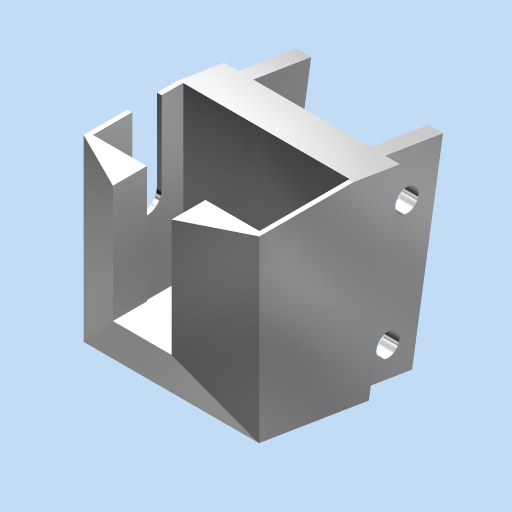
# Autodesk Inventor part: back_mount
Saved by Autodesk Inventor 2024 (Build 280153000, 153)
## iProperties
Created: 2024-02-18
Part Number: back_mount
Material: Aluminum 6061
Document SubType Name: Modeling
Designer: Monesh Ponduri
Density: 2.71 g/cm^3
Appearance: Aluminum - Flat
Author: Monesh Ponduri
## iProperties of the stored document back_mount_3DPrint.ipt
Created: 2024-02-20
Part Number: back_mount_3DPrint
Material: Generic
Document SubType Name: Modeling
Designer: mones
Density: 1 g/cm^3
Appearance: Default
Author: mones
Autodesk Inventor part; units mm, degrees
ref_plane "YZ Plane Vertical Spine" through (0, 0, 0) normal (1, 0, 0) x (0, 1, 0)
ref_plane "XZ Plane Horizontal" through (0, 0, 0) normal (0, 1, 0) x (-1, 0, 0)
ref_plane "XY Plane Vertical Span" through (0, 0, 0) normal (0, 0, 1) x (1, 0, 0)
sketch "Sketch1" plane through (0, 0, 0) normal (1, 0, 0) x (0, 1, 0)
  circle A0 centre (9.6489, 11.4476) radius 2.4892
  line L0 (2.3561, 6.2073) -> (18.2812, 3.5994)
  line L1 (33.7025, 135.9395) -> (135.3025, 135.9395) construction
  line L2 (21.99, 26.2473) -> (-14.84, 26.2473)
  line L3 (4.4085, 18.7403) -> (-20.6576, 22.8451)
  line L4 (-20.6576, 22.8451) -> (-22.71, 10.312)
  line L5 (-22.71, 10.312) -> (2.3561, 6.2073)
  circle A1 centre (-15.4173, 15.5524) radius 2.4892
  line L6 (-14.84, 26.2473) -> (-14.84, 46.5673)
  line L7 (-20.6576, 22.8451) -> (-16.7225, 46.8756)
  line L8 (-16.7225, 46.8756) -> (-14.84, 46.5673)
  line L9 (21.99, 26.2473) -> (18.2812, 3.5994)
  line L10 (20.3336, 16.1325) -> (4.4085, 18.7403)
  dimension "d11" = 12.7
  dimension "d13" = 4.9784
  dimension "d14" = 20.32
  constraints: 22 end point, 3 perpendicular, 2 centre point, 1 horizontal, 1 point on line, 1 vertical
  measures "d11" distance of L3.end L4.end
  measures "d13" diameter of A1
  measures "d14" distance of L2.end L6.end
extrude "Extrusion1" add sketch "Sketch1" along normal blind 3.175
sketch "Sketch2" plane through (0, 0, 0) normal (-1, 0, 0) x (0, 0, 1)
  line L0 (26.2473, 21.99) -> (26.2473, -14.84) projected
  line L1 (3.5994, 18.2812) -> (26.2473, 21.99) projected
  line L2 (26.2473, -14.84) -> (46.5673, -14.84) projected
  line L3 (46.8756, -16.7225) -> (10.312, -22.71) projected
  line L4 (16.1325, 20.3336) -> (22.8451, -20.6576)
  line L5 (16.1325, 20.3336) -> (26.2473, 21.99)
  line L6 (26.2473, 21.5334) -> (26.2473, -14.84)
  line L7 (26.2473, -14.84) -> (46.5673, -14.84)
  line L8 (46.5673, -14.84) -> (46.8756, -16.7225)
  line L9 (46.8756, -16.7225) -> (22.8451, -20.6576)
  constraints: 12 end point, 4 collinear, 3 point on line, 2 perpendicular
extrude "Extrusion2" add sketch "Sketch2" along normal blind 25.4
sketch "Sketch3" plane through (-25.4, 0, 0) normal (-1, 0, 0) x (0, 0, 1)
  line L0 (26.2473, -14.84) -> (26.2473, 21.99) projected
  line L1 (3.5994, 18.2812) -> (16.1325, 20.3336) projected
  line L2 (26.2473, 21.99) -> (16.1325, 20.3336) projected
  line L3 (46.5673, -14.84) -> (26.2473, -14.84) projected
  line L4 (46.8756, -16.7225) -> (46.5673, -14.84) projected
  line L5 (22.8451, -20.6576) -> (46.8756, -16.7225) projected
  line L6 (22.8451, -20.6576) -> (10.312, -22.71) projected
  line L7 (10.312, -22.71) -> (3.5994, 18.2812) projected
  circle A0 centre (15.5524, -15.4173) radius 2.4892 projected
  circle A1 centre (11.4476, 9.6489) radius 2.4892 projected
extrude "Extrusion3" add sketch "Sketch3" along normal blind 3.175
sketch "Sketch4" plane through (-28.575, 0, 0) normal (-1, 0, 0) x (0, 0, 1)
  line L0 (26.2473, 21.99) -> (3.5994, 18.2812) projected
  line L1 (26.2473, -14.84) -> (26.2473, 21.99) projected
  line L2 (46.5673, -14.84) -> (26.2473, -14.84) projected
  line L3 (46.8756, -16.7225) -> (46.5673, -14.84) projected
  line L4 (10.312, -22.71) -> (46.8756, -16.7225) projected
  line L5 (46.8756, -16.7225) -> (46.5673, -14.84) projected
  line L6 (46.5673, -14.84) -> (26.2473, -14.84) projected
  line L7 (26.2473, -14.84) -> (26.2473, 21.99) projected
  line L8 (26.2473, 21.99) -> (3.5994, 18.2812) projected
  line L9 (3.5994, 18.2812) -> (10.312, -22.71) projected
  line L10 (10.312, -22.71) -> (46.8756, -16.7225) projected
  circle A0 centre (11.4476, 9.6489) radius 2.4892 projected
  circle A1 centre (15.5524, -15.4173) radius 2.4892 projected
  line L11 (16.1325, 20.3336) -> (22.8451, -20.6576)
  line L12 (16.1325, 20.3336) -> (26.2473, 21.99)
  line L13 (26.2473, 21.99) -> (26.2473, -14.84)
  line L14 (46.5673, -14.84) -> (26.2473, -14.84)
  line L15 (46.5673, -14.84) -> (46.8756, -16.7225)
  line L16 (46.8756, -16.7225) -> (22.8451, -20.6576)
  constraints: 12 end point, 4 perpendicular, 2 collinear, 1 point on line
extrude "Extrusion4" add sketch "Sketch4" along normal blind 3.175 contours L1 L2 L3 L4 L11 L0
sketch "Sketch5" plane through (3.175, 0, 0) normal (1, 0, 0) x (0, 0, -1)
  line L0 (-22.8451, -20.6576) -> (-16.1325, 20.3336) projected
  line L1 (-46.8756, -16.7225) -> (-10.312, -22.71) projected
  line L2 (-26.2473, -14.84) -> (-46.5673, -14.84) projected
  line L3 (-26.2473, 21.99) -> (-26.2473, -14.84) projected
  line L4 (-3.5994, 18.2812) -> (-26.2473, 21.99) projected
  line L5 (-26.2473, 21.99) -> (-16.1325, 20.3336)
  line L6 (-16.1325, 20.3336) -> (-22.8451, -20.6576)
  line L7 (-22.8451, -20.6576) -> (-46.8756, -16.7225)
  line L8 (-46.8756, -16.7225) -> (-46.5673, -14.84)
  line L9 (-46.5673, -14.84) -> (-26.2473, -14.84)
  line L10 (-26.2473, -14.84) -> (-26.2473, 21.99)
  constraints: 12 end point, 5 collinear, 1 perpendicular
extrude "Extrusion5" add sketch "Sketch5" along normal blind 3.175
sketch "Sketch6" plane through (-31.75, -14.84, 46.5673) normal (0, 1, 0) x (1, 0, 0)
  line L0 (38.1, 20.32) -> (38.1, 0) projected
  line L1 (0, 0) -> (0, 20.32) projected
  line L2 (0, 20.32) -> (1.27, 20.32)
  line L3 (0, 0) -> (1.27, 0)
  line L4 (1.27, 0) -> (1.27, 20.32)
  line L5 (38.1, 0) -> (38.1, 20.32)
  line L6 (38.1, 20.32) -> (36.83, 20.32)
  line L7 (36.83, 20.32) -> (36.83, 0)
  line L8 (36.83, 0) -> (38.1, 0)
  dimension "d24" = 1.27
  dimension "d25" = 1.27
  dimension "d26" = 1.27
  constraints: 14 end point, 3 perpendicular, 2 horizontal, 1 collinear, 1 point on line
  measures "d24" distance of L1.end L2.end
  measures "d25" distance of L1.start L3.end
  measures "d26" distance of L0.start L6.end
extrude "Extrusion6" add sketch "Sketch6" along normal blind 36.83
sketch "Sketch7" plane through (-30.48, -14.84, 26.2473) normal (0, 1, 0) x (1, 0, 0)
  line L0 (0, -20.32) -> (35.56, -20.32) projected
  line L1 (0, -19.05) -> (35.56, -19.05)
  line L2 (0, -20.32) -> (35.56, -20.32)
  line L3 (35.56, -19.05) -> (35.56, -20.32)
  line L4 (0, -19.05) -> (0, -20.32)
  dimension "d29" = 1.27
  constraints: 8 end point, 3 equal length, 1 perpendicular
  measures "d29" distance between parallel lines of L0 L1
extrude "Extrusion7" add sketch "Sketch7" along normal blind 11.43
sketch "Sketch8" plane through (-30.48, -14.84, 26.2473) normal (1, 0, 0) x (0, 0, -1)
  line L0 (-20.32, 11.43) -> (-20.32, 36.83) projected
  line L1 (-19.05, 11.43) -> (-19.05, 36.83)
  line L2 (-19.05, 36.83) -> (-20.32, 36.83)
  line L3 (-19.05, 11.43) -> (-20.32, 11.43)
  line L4 (-20.32, 11.43) -> (-20.32, 36.83)
  dimension "d32" = 1.27
  constraints: 8 end point, 3 equal length, 1 horizontal
  measures "d32" distance between parallel lines of L0 L1
extrude "Extrusion8" add sketch "Sketch8" along normal blind 11.43
sketch "Sketch9" plane through (5.08, -14.84, 26.2473) normal (-1, 0, 0) x (0, 0, 1)
  line L0 (20.32, 11.43) -> (20.32, 36.83) projected
  line L1 (19.0567, 11.43) -> (19.0567, 36.83)
  line L2 (19.0567, 36.83) -> (20.32, 36.83)
  line L3 (20.32, 36.83) -> (20.32, 11.43)
  line L4 (20.32, 11.43) -> (19.0567, 11.43)
  constraints: 8 end point, 2 equal length, 1 horizontal, 1 perpendicular
extrude "Extrusion9" add sketch "Sketch9" along normal blind 11.43
sketch "Sketch10" plane through (-31.75, 0, 0) normal (-1, 0, 0) x (0, 0, 1)
  line L0 (46.5673, -14.84) -> (46.5673, 21.99) projected
  line L1 (22.8451, -20.6576) -> (46.8756, -16.7225) projected
  line L2 (46.5673, -14.84) -> (46.5673, -16.773)
  line L3 (46.5673, -16.773) -> (47.6603, -17.0438)
  line L4 (47.6603, -17.0438) -> (46.5673, -14.84)
  constraints: 6 end point, 1 point on line, 1 vertical
extrude "Extrusion10" cut sketch "Sketch10" against normal blind 50.8
thicken "Thicken1" operation add thickness 6.35 both sides no extend neighbours no toward (0, 0, 1) faces at (-10.5833, -12.3187, 46.5673)
sketch "Sketch11" plane through (-31.75, 0, 0) normal (-1, 0, 0) x (0, 0, 1)
  line L0 (22.8451, -20.6576) -> (46.5673, -16.773) projected
  line L1 (46.5673, -16.773) -> (55.5301, -15.3053)
  line L2 (55.5301, -15.3053) -> (55.5301, -20.6762)
  line L3 (55.5301, -20.6762) -> (46.5673, -16.773)
  constraints: 6 end point, 1 vertical
extrude "Extrusion11" cut sketch "Sketch11" against normal blind 50.8
chamfer "Chamfer1" distance 6.35 distance2 12.7 1 edges at (-31.75, 3.1284, 52.9173) measured on face at (-31.75, -4.8003, 34.0032)
chamfer "Chamfer2" distance 6.35 distance2 12.7 1 edges at (6.35, 3.1284, 52.9173) measured on face at (6.35, -4.8003, 34.0032)
chamfer "Chamfer3" distance 6.35 distance2 12.319 1 edges at (-12.7, -15.7331, 52.9173) measured on face at (-14.8167, -19.0161, 32.8692)
sketch "Sketch13" plane through (-31.75, 0, 0) normal (-1, 0, 0) x (0, 0, 1)
  line L0 (26.2473, 21.99) -> (46.5673, 21.99) projected
  line L1 (37.0423, 21.99) -> (33.8673, 21.99)
  line L2 (30.6923, 21.99) -> (30.6923, 4.21)
  line L3 (37.0423, 4.21) -> (37.0423, 21.99)
  line L4 (37.0423, 21.99) -> (30.6923, 21.99)
  arc A0 (30.6923, 4.21) -> (37.0423, 4.21) centre (33.8673, 4.21) ccw
  point P0 (30.6923, 4.21)
  constraints: 8 end point, 2 point on circle, 1 centre point, 1 parallel, 1 point on line
extrude "Extrusion12" cut sketch "Sketch13" against normal blind 25.4
sketch "Sketch14" plane through (-30.48, -14.84, 26.2473) normal (0, 1, 0) x (1, 0, 0)
  line L0 (0, -19.05) -> (35.56, -19.05) projected
  line L1 (35.56, -19.05) -> (35.56, 0) projected
  line L2 (0, 0) -> (35.56, 0) projected
  line L3 (0, 0) -> (0, -19.05) projected
  line L4 (35.814, 0.254) -> (35.814, -19.304)
  line L5 (35.814, -19.304) -> (-0.254, -19.304)
  line L6 (-0.254, -19.304) -> (-0.254, 0.254)
  line L7 (-0.254, 0.254) -> (35.814, 0.254)
  dimension "d57" = 0.254
  constraints: 8 end point, 3 other
  measures "d57" distance between parallel lines of L2 L7
extrude "Extrusion13" cut sketch "Sketch14" along normal blind 50.8 contours L3 L2 L1 L0 | L4 L5 L6 L7
sketch "Sketch15" plane through (-30.734, -14.84, 45.5513) normal (0, 1, 0) x (1, 0, 0)
  line L0 (0, 19.558) -> (0, 0) projected
  line L1 (0, 0) -> (36.068, 0) projected
  line L2 (36.068, 0) -> (36.068, 19.558) projected
  line L3 (36.068, 19.558) -> (0, 19.558) projected
  line L4 (0, 9.779) -> (36.068, 9.779)
  line L5 (18.034, 0) -> (18.034, 19.558)
  circle A0 centre (18.034, 9.779) radius 6.35
  dimension "d60" = 12.7
  constraints: 5 midpoint, 4 end point, 1 centre point
  measures "d60" diameter of A0
extrude "Extrusion14" cut sketch "Sketch15" against normal blind 50.8 contours A0 L5 L4 | L4 L5 A0 | A0 L4 L5 | L4 A0 L5
body "Solid1"
